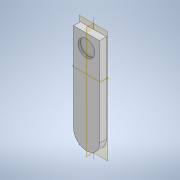
# Autodesk Inventor part: Push
Saved by Autodesk Inventor 2021 (Build 250183000, 183)
## iProperties
Created: 2022-11-29
Part Number: Push
Material: Generisch
Document SubType Name: Modeling
Designer: Elian
Density: 1 g/cm^3
Appearance: Vorgabe
Author: Elian
Autodesk Inventor part; units mm, degrees
sketch "Skizze1" plane through (0, 0, 0) normal (0, 0, 1) x (1, 0, 0)
  line L0 (19, 51.5252) -> (-19, 51.5252)
  line L1 (-19, 51.5252) -> (-19, -78.4748)
  line L2 (-19, -78.4748) -> (19, -78.4748)
  line L3 (19, -78.4748) -> (19, 51.5252)
  line L4 (0, -127.2748) -> (0, 81.3252) projected
  circle A0 centre (0, -78.4748) radius 19
  point P0 (0, 0)
  dimension "d0" = 130
  dimension "d1" = 38
  constraints: 8 end point, 2 parallel, 1 horizontal, 1 midpoint, 1 perpendicular, 1 point on line, 4 other
  measures "d0" distance of L0.end L1.end
  measures "d1" distance of L0.start L0.end
extrude "Extrusion1" add sketch "Skizze1" along normal blind 10
sketch "Skizze2" plane through (0, 0, 10) normal (0, 0, 1) x (1, 0, 0)
  circle A0 centre (0, 32.5252) radius 12
  line L0 (19, 51.5252) -> (-19, 51.5252) projected
  point P0 (0, 0)
  dimension "d4" = 24
  dimension "d5" = 19
  constraints: 1 centre point
  measures "d4" diameter of A0
  measures "d5" distance from line of L0 A0.centre
extrude "Extrusion2" cut sketch "Skizze2" against normal blind 3
